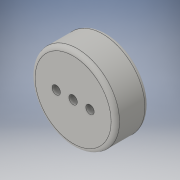
# Autodesk Inventor part: friction-fit
Saved by Autodesk Inventor 2016 (Build 200138000, 138)
## iProperties
Created: 2015-08-19
Part Number: friction-fit
Material: Generic
Document SubType Name: Modeling
Designer: chdsbd
Density: 1 g/cm^3
Appearance: Default
Author: chdsbd
Autodesk Inventor part; units mm, degrees
ref_plane "YZ Plane" through (0, 0, 0) normal (1, 0, 0) x (0, 1, 0)
ref_plane "XZ Plane" through (0, 0, 0) normal (0, 1, 0) x (-1, 0, 0)
ref_plane "XY Plane" through (0, 0, 0) normal (0, 0, 1) x (1, 0, 0)
sketch "Sketch1" plane through (0, 0, 0) normal (0, 0, 1) x (1, 0, 0)
  circle A0 centre (0, 0) radius 25.4
  circle A1 centre (0, 0) radius 31.75
  dimension "d1" = 50.8
  dimension "d2" = 6.35
  constraints: 2 centre point, 2 coincident
  measures "d1" diameter of A0
  measures "d2" radial gap between concentric circles of A1 A0
extrude "Ring" add sketch "Sketch1" against normal blind 19.05
extrude "Back" add sketch "Sketch1" along normal blind 6.35 contours A0 | A1
sketch "Sketch2" plane through (0, 0, 6.35) normal (0, 0, 1) x (1, 0, 0)
  circle A0 centre (0, 0) radius 3.175
  circle A1 centre (-12.7, 0) radius 3.175
  circle A2 centre (12.7, 0) radius 3.175
  line L0 (-12.7, 0) -> (12.7, 0) construction
  dimension "d7" = 6.35
  dimension "d8" = 12.7
  dimension "d11" = 12.7
  constraints: 3 centre point, 2 end point, 2 equal radius, 1 coincident, 1 horizontal, 1 midpoint
  measures "d7" diameter of A0
  measures "d8" distance of point (0, 0) L0.start
  measures "d11" distance of L0.end point (0, 0)
extrude "Holes" cut sketch "Sketch2" against normal through all
fillet "Fillets" radius 3.175 3 edges at (-31.75, 0, 6.35) (-31.75, 0, -19.05) (-25.4, 0, -19.05)
body "Solid1"
